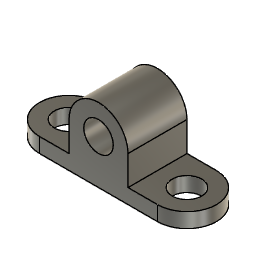
A4 (Autodesk Fusion 360 design; units mm, degrees)
Autodesk Fusion 360 part; units mm, degrees
note: some values were not read from the file. Chosen so that the rebuilt part matches the saved one: which pieces of a blend or face edit are solid.
sketch "Sketch1" plane through (0, 0, 0) normal (0, 0, 1) x (1, 0, 0)
  line L0 (-60, 30) -> (60, 30)
  line L1 (60, 30) -> (60, -10)
  line L2 (60, -10) -> (-60, -10)
  line L3 (-60, -10) -> (-60, 30)
  dimension "d1" = 120
  dimension "d2" = 40
  constraint horizontal L0
  constraint vertical L1
  constraint horizontal L2
  constraint vertical L3
  measures "d1" distance of L0.start L0.end
  measures "d2" distance of L0.start L2.end
extrude "Extrude1" add sketch "Sketch1" along normal blind 10
fillet "Fillet1" radius 20 1 faces at (60, 16.6667, 3.3333)
fillet "Fillet2" radius 20 1 faces at (-60, 3.3333, 3.3333)
sketch "Sketch2" plane through (0, 0, 10) normal (0, 0, 1) x (-1, 0, 0)
  arc A0 (40, -30) -> (40, 10) centre (40, -10) ccw
  line L0 (40, 10) -> (-40, 10)
  arc A1 (-40, 10) -> (-40, -30) centre (-40, -10) ccw
  line L1 (-40, -30) -> (40, -30)
  circle A2 centre (40, -10) radius 10
  circle A3 centre (-40, -10) radius 10
  dimension "d9" = 20
  dimension "d10" = 20
  constraint concentric A0 A2
  constraint concentric A1 A3
  measures "d9" diameter of A2
  measures "d10" diameter of A3
hole "Hole1" at (-40, 10, 10) direction (0, 0, -1) diameter 20 depth 50 tip angle 118
sketch "Sketch3" plane through (0, 0, 10) normal (0, 0, 1) x (-1, 0, 0)
  circle A0 centre (40, -10) radius 10
  arc A1 (40, -30) -> (40, 10) centre (40, -10) ccw
  line L0 (40, 10) -> (-40, 10)
  arc A2 (-40, 10) -> (-40, -30) centre (-40, -10) ccw
  line L1 (-40, -30) -> (40, -30)
  circle A3 centre (-40, -10) radius 10
  dimension "d14" = 20
  constraint concentric A2 A3
  measures "d14" diameter of A3
hole "Hole2" at (40, 10, 10) direction (0, 0, -1) diameter 20 depth 50 tip angle 118
sketch "Sketch4" plane through (0, 0, 10) normal (0, 0, 1) x (-1, 0, 0)
  circle A0 centre (-40, -10) radius 10
  circle A1 centre (40, -10) radius 10
  arc A2 (40, -30) -> (40, 10) centre (40, -10) ccw
  line L0 (40, 10) -> (-40, 10)
  arc A3 (-40, 10) -> (-40, -30) centre (-40, -10) ccw
  line L1 (-40, -30) -> (40, -30)
  line L2 (0, -30) -> (-20, -30)
  line L3 (-20, -30) -> (-20, 10)
  line L4 (-20, 10) -> (0, 10)
  line L5 (0, 10) -> (0, -30)
  line L6 (0, -30) -> (20, -30)
  line L7 (20, -30) -> (20, 10)
  line L8 (20, 10) -> (0, 10)
  line L9 (0, 10) -> (0, -30)
  dimension "d18" = 20
  dimension "d19" = 20
  constraint horizontal L2
  constraint vertical L3
  constraint horizontal L4
  constraint vertical L5
  constraint coincident L0 L3.end
  constraint midpoint L1 L2.start
  constraint horizontal L6
  constraint vertical L7
  constraint horizontal L8
  constraint vertical L9
  constraint coincident L0 L7.end
  measures "d18" distance of L2.start L2.end
  measures "d19" distance of L2.start L6.end
extrude "Extrude2" add sketch "Sketch4" along normal blind 40 contours L0 L1 L5 L6 L7 L8 L9 | L0 L1 L2 L3 L4 L5 L9
fillet "Fillet3" radius 20 2 edges at (-20, 10, 50) (20, 10, 50)
sketch "Sketch5" plane through (0, -10, 0) normal (0, -1, 0) x (1, 0, 0)
  arc A0 (20, 30) -> (-20, 30) centre (0, 30) ccw
  line L0 (-20, 30) -> (-20, 10)
  line L1 (-20, 10) -> (-40, 10)
  line L2 (-40, 10) -> (-40, 0)
  line L3 (-40, 0) -> (40, 0)
  line L4 (40, 0) -> (40, 10)
  line L5 (40, 10) -> (20, 10)
  line L6 (20, 10) -> (20, 30)
  circle A1 centre (0, 30) radius 10
  dimension "d24" = 20
  constraint concentric A0 A1
  measures "d24" diameter of A1
hole "Hole3" at (0, -10, 30) direction (0, 1, 0) diameter 20 depth 50 tip angle 118
